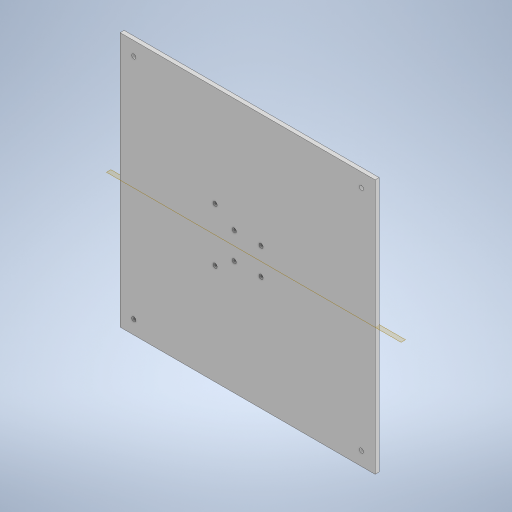
# Autodesk Inventor part: print bed base
Saved by Autodesk Inventor 2023.1 (Build 271208000, 208)
## iProperties
Created: 2022-10-30
Part Number: print bed base
Material: Generic
Document SubType Name: Modeling
Designer: nicol
Density: 1 g/cm^3
Appearance: Default
Author: nicol
Autodesk Inventor part; units mm, degrees
ref_plane "YZ Plane" through (0, 0, 0) normal (1, 0, 0) x (0, 1, 0)
ref_plane "XZ Plane" through (0, 0, 0) normal (0, 1, 0) x (-1, 0, 0)
ref_plane "XY Plane" through (0, 0, 0) normal (0, 0, 1) x (1, 0, 0)
sketch "Sketch1" plane through (0, 0, 0) normal (0, 0, 1) x (1, 0, 0)
  line L0 (0, 0) -> (190.5, 0)
  line L1 (190.5, 0) -> (190.5, 190.5)
  line L2 (190.5, 190.5) -> (0, 190.5)
  line L3 (0, 190.5) -> (0, 0)
  dimension "d0" = 190.5
  dimension "d1" = 190.5
  constraints: 8 end point, 2 parallel, 1 horizontal, 1 perpendicular
  measures "d0" distance of L2.end L1.end
  measures "d1" distance of L1.end L0.end
extrude "Extrusion1" add sketch "Sketch1" along normal blind 3
ref_plane "Work Plane1" through (0, 95.25, 0) normal (0, 1, 0) x (1, 0, 0)
sketch "Sketch2" plane through (0, 0, 3) normal (0, 0, 1) x (1, 0, 0)
  line L0 (0, 190.5) -> (0, 0) projected
  line L1 (190.5, 0) -> (190.5, 190.5) projected
  line L2 (0, 0) -> (190.5, 0) projected
  line L3 (190.5, 190.5) -> (0, 190.5) projected
  line L4 (32.6, 104.25) -> (56.6, 104.25) construction
  line L5 (133.9, 104.25) -> (157.9, 104.25) construction
  line L6 (85.25, 105.25) -> (105.25, 105.25) construction
  line L7 (105.25, 105.25) -> (105.25, 85.25) construction
  line L8 (105.25, 85.25) -> (85.25, 85.25) construction
  line L9 (85.25, 85.25) -> (85.25, 105.25) construction
  line L10 (70.925, 115.25) -> (70.925, 75.25) construction
  point P0 (10.25, 180.25)
  point P1 (180.25, 180.25)
  point P2 (180.25, 10.25)
  point P3 (10.25, 10.25)
  point P4 (32.6, 86.25)
  point P5 (56.6, 86.25)
  point P6 (133.9, 86.25)
  point P7 (157.9, 86.25)
  point P8 (44.6, 104.25)
  point P9 (145.9, 104.25)
  point P10 (95.25, 105.25)
  point P11 (95.25, 190.5)
  point P12 (105.25, 95.25)
  point P13 (190.5, 95.25)
  point P14 (70.925, 95.25)
  point P15 (0, 95.25)
  dimension "d4" = 170
  dimension "d5" = 170
  dimension "d6" = 10.25
  dimension "d7" = 10.25
  dimension "d8" = 10.25
  dimension "d9" = 10.25
  dimension "d17" = 24
  dimension "d18" = 18
  dimension "d19" = 18
  dimension "d20" = 24
  dimension "d21" = 101.3
  dimension "d22" = 32.6
  dimension "d23" = 32.6
  dimension "d24" = 86.25
  dimension "d25" = 86.25
  dimension "d33" = 20
  dimension "d34" = 40
  dimension "d35" = 14.325
  dimension "d36" = 14.325
  constraints: 14 end point, 8 horizontal alignment, 8 midpoint, 7 vertical alignment, 4 coincident, 3 horizontal, 2 parallel, 2 perpendicular, 1 collinear, 1 vertical
  measures "d4" distance of point (10.25, 180.25) point (180.25, 180.25)
  measures "d5" distance of point (180.25, 10.25) point (180.25, 180.25)
  measures "d6" distance from line of L0 point (10.25, 180.25)
  measures "d7" distance from line of L1 point (180.25, 180.25)
  measures "d8" distance from line of L2 point (180.25, 10.25)
  measures "d9" distance from line of L3 point (180.25, 180.25)
  measures "d17" distance of L5.end L5.start
  measures "d18" distance of point (157.9, 86.25) L5.end
  measures "d19" distance of point (56.6, 86.25) L4.end
  measures "d20" distance of L4.start L4.end
  measures "d21" distance of point (44.6, 104.25) point (145.9, 104.25)
  measures "d22" distance from line of L1 point (157.9, 86.25)
  measures "d23" distance from line of L0 point (32.6, 86.25)
  measures "d24" distance from line of L3 L5.end
  measures "d25" distance from line of L2 point (157.9, 86.25)
  measures "d33" distance of L6.start L6.end
  measures "d34" distance of L10.start L10.end
  measures "d35" distance from line of point (85.25, 105.25) L10
  measures "d36" distance from line of L4.end L10
hole "Hole1" at (10.25, 180.25, 3) at (180.25, 180.25, 3) at (180.25, 10.25, 3) at (10.25, 10.25, 3) at (85.25, 105.25, 3) at (105.25, 105.25, 3) at (105.25, 85.25, 3) at (85.25, 85.25, 3) at (70.925, 115.25, 3) at (70.925, 75.25, 3) direction (0, 0, -1) diameter 3.2 end through all
equation "\"d5\" = d4"
equation "\"d6\" = d7"
equation "\"d8\" = d9"
equation "\"d19\" = d18"
equation "\"d20\" = d17"
equation "\"d22\" = d23"
equation "\"d24\" = d25"
equation "\"d35\" = d36"
body "Solid1"
